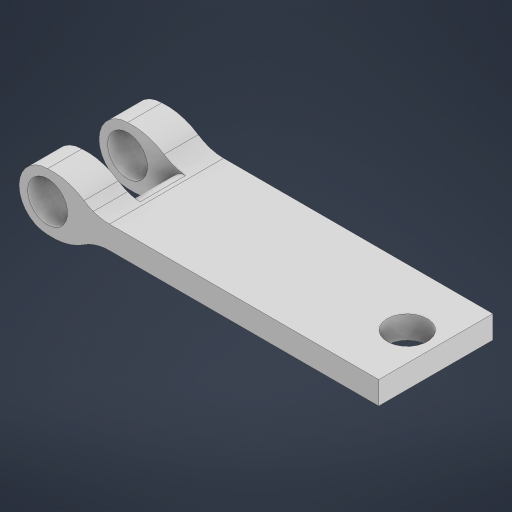
# Autodesk Inventor part: lamp_p1
Saved by Autodesk Inventor 2024.4 (Build 284460000, 460)
## iProperties
Created: 2026-05-15
Part Number: lamp_p1
Material: Ogólny
Document SubType Name: Modeling
Designer: User
Density: 1 g/cm^3
Appearance: Domyślna
Author: User
Autodesk Inventor part; units mm, degrees
ref_plane "YZ Plane" through (0, 0, 0) normal (1, 0, 0) x (0, 1, 0)
ref_plane "XZ Plane" through (0, 0, 0) normal (0, 1, 0) x (-1, 0, 0)
ref_plane "XY Plane" through (0, 0, 0) normal (0, 0, 1) x (1, 0, 0)
sketch "Szkic1" plane through (0, 0, 0) normal (0, 1, 0) x (-1, 0, 0)
  line L0 (-2.5, 5) -> (2.5, 5)
  line L1 (2.5, 5) -> (2.5, -5)
  line L2 (2.5, -5) -> (-2.5, -5)
  line L3 (-2.5, -5) -> (-2.5, 5)
  line L4 (-2.5, 5) -> (2.5, -5) construction
  line L5 (2.5, 5) -> (-2.5, -5) construction
  circle A0 centre (0, 0) radius 1.75
  line L6 (2.5, 5) -> (22.5, 5)
  line L7 (22.5, 5) -> (22.5, -5)
  line L8 (22.5, -5) -> (2.5, -5)
  line L9 (2.5, -5) -> (2.5, 5)
  dimension "d0" = 5
  dimension "d1" = 10
  dimension "d2" = 3.5
  dimension "d3" = 20
  dimension "d4" = 10
  constraints: 20 end point, 4 parallel, 2 horizontal, 2 midpoint, 2 perpendicular, 1 centre point, 1 coincident
  measures "d0" distance of L1.end L2.end
  measures "d1" distance of L0.end L1.end
  measures "d2" diameter of A0
  measures "d3" distance of L7.end L8.end
  measures "d4" distance of L6.end L7.end
extrude "Wyciągnięcie proste1" add sketch "Szkic1" along normal blind 2
sketch "Szkic2" plane through (2.5, 0, -5) normal (0, 0, -1) x (-1, 0, 0)
  line L0 (25, 0) -> (25, 2) projected
  line L1 (25, 1) -> (29, 1)
  line L2 (25, 1) -> (29, 1) construction
  circle A0 centre (29, 1) radius 1.75
  circle A1 centre (29, 1) radius 2.5
  line L3 (29, 3.5) -> (29, 3.5)
  line L4 (29, -1.5) -> (29, -1.5)
  arc A2 (29, 3.5) -> (25, 2) centre (28.5874, -1.4829) ccw
  arc A3 (25, 0) -> (29, -1.5) centre (28.5874, 3.4829) ccw
  point P0 (2.5, 0)
  point P1 (29, 3.5)
  point P2 (29, -1.5)
  dimension "d10" = 4
  dimension "d11" = 0
  dimension "d12" = 3.5
  dimension "d13" = 5
  dimension "d14" = 0
  dimension "d15" = 0
  dimension "d16" = 5
  dimension "d17" = 5
  constraints: 8 end point, 6 point on circle, 4 centre point, 2 coincident, 2 horizontal, 2 vertical, 1 collinear, 1 midpoint
  measures "d10" distance of L1.start L1.end
  measures "d11" distance between parallel lines of L1 L2
  measures "d12" diameter of A0
  measures "d13" diameter of A1
  measures "d14" distance of L3.start L3.end
  measures "d15" distance of L4.start L4.end
  measures "d16" radius of A2
  measures "d17" radius of A3
extrude "Wyciągnięcie proste2" add sketch "Szkic2" against normal blind 3
ref_plane "Płaszczyzna konstrukcyjna1" through (2.5, 0, 0) normal (0, 0, -1) x (-1, 0, 0)
mirror "Odbij1" about plane through (2.5, 0, 0) normal (0, 0, -1) of "Wyciągnięcie proste2"
fillet "Zaokrąglenie1" radius 4 4 edges at (-22.5, 2, -3.5) (-22.5, 2, 3.5) (-22.5, 0, -3.5) (-22.5, 0, 3.5)
fillet "Zaokrąglenie2" radius 1 2 edges at (-22.5, -0.258, 0) (-22.5, 2.258, 0)
